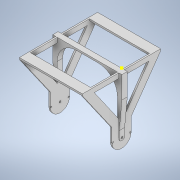
# Autodesk Inventor part: bottom_gimbal_ring_3
Saved by Autodesk Inventor 2022 (Build 260153000, 153)
## iProperties
Created: 2022-03-15
Part Number: bottom_gimbal_ring_3
Material: Generic
Document SubType Name: Modeling
Designer: kylem
Density: 1 g/cm^3
Appearance: Default
Author: kylem
Autodesk Inventor part; units mm, degrees
ref_plane "YZ Plane" through (0, 0, 0) normal (1, 0, 0) x (0, 1, 0)
ref_plane "XZ Plane" through (0, 0, 0) normal (0, 1, 0) x (-1, 0, 0)
ref_plane "XY Plane" through (0, 0, 0) normal (0, 0, 1) x (1, 0, 0)
sketch "Sketch1" plane through (0, 0, 0) normal (0, 1, 0) x (-1, 0, 0)
  circle A0 centre (0, 0) radius 16.375
  dimension "d0" = 32.75
  constraints: 1 centre point, 1 coincident
  measures "d0" diameter of A0
extrude "Extrusion1" add sketch "Sketch1" along normal blind 3
sketch "Sketch2" plane through (0, 3, 0) normal (0, 1, 0) x (1, 0, 0)
  circle A0 centre (0, 0) radius 4.75
  dimension "d3" = 9.5
  constraints: 1 centre point, 1 coincident
  measures "d3" diameter of A0
extrude "Extrusion2" add sketch "Sketch2" along normal blind 14
chamfer "Chamfer1" distance 1 angle 45 1 edges at (-4.75, 17, 0)
sketch "Sketch3" plane through (0, 3, 0) normal (0, 1, 0) x (1, 0, 0)
  circle A0 centre (0, 0) radius 15.5
  circle A1 centre (0, 0) radius 16.375
  line L0 (0, 0) -> (0, 16.375)
  circle A2 centre (0, 0) radius 16.375 projected
  line L1 (0, 0) -> (16.375, 0)
  point P0 (15.5, 0)
  point P1 (0, 15.5)
  dimension "d9" = 31
  dimension "d26" = 32.75
  constraints: 4 end point, 2 centre point, 2 coincident, 2 point on circle, 1 horizontal
  measures "d9" diameter of A0
  measures "d26" diameter of A1
extrude "Extrusion3" add sketch "Sketch3" along normal blind 13.5 contours A0 L0 A1 L1 picked at (14.8943, 5.8246)
sketch "Sketch4" plane through (0, 16.5, 0) normal (0, 1, 0) x (1, 0, 0)
  arc A0 (-10.8502, -12.2644) -> (-12.2644, -10.8502) centre (0, 0) ccw
  circle A1 centre (0, 0) radius 3.75 projected
  line L0 (0, 16.375) -> (0, 15.5) projected
  arc A2 (-10.2302, -11.6444) -> (-11.6444, -10.2302) centre (0, 0) ccw
  line L1 (0, 0) -> (-0.7071, 0.7071)
  line L2 (0, 0) -> (1, 0) construction
  line L3 (-0.7071, 0.7071) -> (0.7071, -0.7071)
  line L4 (1.0882, -0.326) -> (-18.1603, -19.5746)
  line L5 (-0.7071, 0.7071) -> (-13.3956, -11.9813)
  line L6 (-13.3956, -11.9813) -> (-11.0324, -14.3445)
  line L7 (-10.2302, -11.6444) -> (-7.7553, -14.1193)
  line L8 (-10.2302, -11.6444) -> (-6.7302, -11.6444) construction
  line L9 (-7.9511, -14.3151) -> (-11.998, -18.3619)
  line L10 (-14.4448, -7.7128) -> (-18.1483, -4.0093)
  line L11 (-11.6444, -10.2302) -> (-4.6444, -10.2302) construction
  line L12 (-18.1483, -4.0093) -> (-22.391, -8.252)
  line L13 (-18.1483, -4.0093) -> (-12.1483, -4.0093) construction
  line L14 (-13.3956, -11.9813) -> (-20.1314, -18.7172)
  line L15 (-18.1603, -19.5746) -> (-18.1603, -19.5746)
  line L16 (-18.1603, -19.5746) -> (-21.0847, -16.6502)
  line L17 (-22.391, -8.252) -> (-16.0286, -14.6144)
  line L18 (-14.4729, -15.8871) -> (-11.998, -18.3619)
  dimension "d12" = 1
  dimension "d13" = 135
  dimension "d14" = 2
  dimension "d15" = 0
  dimension "d16" = 3.5
  dimension "d17" = 45
  dimension "d18" = 6
  dimension "d19" = 90
  dimension "d20" = 9
  dimension "d21" = 135
  dimension "d22" = 6
  dimension "d23" = 135
  dimension "d29" = 16.375
  dimension "d30" = 2
  dimension "d31" = 3.5
  constraints: 36 end point, 9 perpendicular, 7 point on circle, 7 point on line, 4 horizontal, 3 equal length, 2 centre point, 2 coincident, 1 collinear
  measures "d12" distance of L1.start L1.end
  measures "d13" angle of L2 L1
  measures "d14" distance of L1.end L3.end
  measures "d15" distance between parallel lines of L3 L1
  measures "d16" distance of L7.start L7.end
  measures "d17" angle of L7 L8
  measures "d18" distance of L7.end L9.end
  measures "d19" angle of L7 L9
  measures "d20" distance of L11.start L10.end
  measures "d21" angle of L11 L10
  measures "d22" distance of L10.end L12.end
  measures "d23" angle of L12 L13
  measures "d29" radius of A0
  measures "d30" distance between parallel lines of L15 L14
  measures "d31" distance between parallel lines of L9 L4
extrude "Extrusion5" add sketch "Sketch4" against normal blind 13 contours L4 A2 L0 A0 | A0 L9 L18 L4 | L0 A2 L5 A0 | L14 L17 L12 L10 A0 L5
sketch "Sketch6" plane through (0, 16.5, 0) normal (0, 1, 0) x (1, 0, 0)
  line L0 (-11.6444, -10.2302) -> (-9.6444, -10.2302) construction
  line L1 (-22.391, -8.252) -> (-16.0286, -14.6144) projected
  line L2 (-16.0286, -14.6144) -> (-17.4428, -13.2001)
  line L3 (-16.0286, -14.6144) -> (-11.6444, -10.2302) projected
  line L4 (-16.0286, -14.6144) -> (-11.6444, -10.2302)
  line L5 (-16.0286, -14.6144) -> (-17.4428, -13.2001)
  line L6 (-16.0286, -14.6144) -> (-14.0286, -14.6144) construction
  line L7 (-17.4428, -13.2001) -> (-10.3717, -6.1291)
  line L8 (-10.3717, -6.1291) -> (-8.2504, -8.2504)
  line L9 (-10.3717, -6.1291) -> (-7.3717, -6.1291) construction
  line L10 (-8.2504, -8.2504) -> (-15.3215, -15.3215)
  line L11 (-16.0286, -14.6144) -> (-22.391, -8.252) projected
  line L12 (-15.3215, -15.3215) -> (-17.4428, -13.2001)
  line L13 (-8.252, -22.391) -> (-14.6144, -16.0286)
  line L14 (-13.2001, -17.4428) -> (-6.1291, -10.3717)
  line L15 (-6.1291, -10.3717) -> (-8.2504, -8.2504)
  line L16 (-15.3215, -15.3215) -> (-13.2001, -17.4428)
  point P0 (0, 0)
  dimension "d34" = 2
  dimension "d35" = 135
  dimension "d36" = 10
  dimension "d37" = 90
  dimension "d39" = 3
  dimension "d40" = 45
  dimension "d41" = 10
  dimension "d42" = 90
  constraints: 28 end point, 4 symmetric about line, 3 horizontal, 2 collinear, 2 equal length, 2 perpendicular, 2 point on line
  measures "d34" distance of L1.end L2.end
  measures "d35" angle of L6 L5
  measures "d36" distance of L2.end L7.end
  measures "d37" angle of L5 L7
  measures "d39" distance of L7.end L8.end
  measures "d40" angle of L8 L9
  measures "d41" distance of L8.end L10.end
  measures "d42" angle of L8 L10
extrude "Extrusion6" cut sketch "Sketch6" against normal blind 13
sketch "Sketch7" plane through (0, 16.5, 0) normal (0, 1, 0) x (1, 0, 0)
  circle A0 centre (0, 0) radius 3.75 projected
  circle A1 centre (0, 0) radius 16.375
  line L0 (-22.391, -8.252) -> (-12.1273, 2.0117)
  line L1 (-22.391, -8.252) -> (-7.876, -8.252) construction
  line L2 (-18.1483, -4.0093) -> (-14.4448, -7.7128) projected
  line L3 (-18.1483, -4.0093) -> (-14.4448, -7.7128)
  line L4 (-7.9511, -14.3151) -> (-11.998, -18.3619) projected
  line L5 (-11.998, -18.3619) -> (-9.8767, -16.2406)
  line L6 (-9.8767, -16.2406) -> (-5.4147, -15.4539)
  circle A2 centre (0, 0) radius 16.375 projected
  line L7 (-9.8767, -16.2406) -> (-7.9511, -14.3151)
  point P0 (-16.2397, -2.1007)
  dimension "d45" = 45
  dimension "d46" = 3
  dimension "d47" = 145
  constraints: 12 end point, 2 collinear, 1 centre point, 1 coincident, 1 equal length, 1 horizontal, 1 point on circle, 1 point on line
  measures "d45" angle of L1 L0
  measures "d46" distance of L4.end L5.end
  measures "d47" angle of L5 L6
extrude "Extrusion7" add sketch "Sketch7" against normal blind 13 contours L2 L0 A1 | A1 L6 L4
sketch "Sketch8" plane through (0, 16.5, 0) normal (0, 1, 0) x (1, 0, 0)
  circle A0 centre (0, 0) radius 3.75 projected
  line L0 (-13.0586, -17.3013) -> (-8.6316, -12.8742) projected
  circle A1 centre (0, 0) radius 15.5
  circle A2 centre (0, 0) radius 16.375
  arc A3 (-8.6316, -12.8742) -> (-12.8742, -8.6316) centre (0, 0) ccw projected
  circle A4 centre (0, 0) radius 27.7287
  constraints: 3 centre point, 3 coincident, 1 point on circle
extrude "Extrusion8" cut sketch "Sketch8" against normal blind 7 contours A4
chamfer "Chamfer2" distance 6 angle 45 1 edges at (-4.75, 3, 0)
sketch "Sketch9" plane through (-11.998, 3.5, 18.3619) normal (0.7071068, 0, 0.7071068) x (0.7071068, 0, -0.7071068)
  line L0 (-0.2001, 6) -> (8.4991, 6) projected
  line L1 (-0.2001, 6) -> (2.7999, 6)
  line L2 (2.7999, 6) -> (2.7999, 3)
  line L3 (3, 0) -> (3, 6) projected
  circle A0 centre (2.7999, 3) radius 1.35
  point P0 (21.4677, -3.5)
  dimension "d55" = 3
  dimension "d56" = 3
  dimension "d57" = 90
  dimension "d58" = 2.7
  constraints: 4 end point, 1 centre point, 1 coincident, 1 parallel, 1 point on line
  measures "d55" distance of L0.start L1.end
  measures "d56" distance of L1.end L2.end
  measures "d57" angle of L1 L2
  measures "d58" diameter of A0
extrude "Extrusion9" cut sketch "Sketch9" along normal mid plane 50 contours A0 L3 | A0 L3
sketch "Sketch10" plane through (-8.6316, 3.5, 12.8742) normal (-0.7071068, 0, -0.7071068) x (-0.7071068, 0, 0.7071068)
  circle A0 centre (3.4609, 3) radius 1.35 projected
  circle A1 centre (3.4609, 3) radius 1.6
  point P0 (-15.2069, -3.5)
  dimension "d61" = 3.2
  constraints: 1 centre point, 1 coincident
  measures "d61" diameter of A1
extrude "Extrusion10" cut sketch "Sketch10" against normal blind 50 contours A0 | A1
sketch "Sketch11" plane through (-11.998, 3.5, 18.3619) normal (0.7071068, 0, 0.7071068) x (0.7071068, 0, -0.7071068)
  arc A0 (3, 1.4126) -> (3, 4.5874) centre (2.7999, 3) ccw projected
  circle A1 centre (2.7999, 3) radius 3
  line L0 (3, 0) -> (0, 0) projected
  point P0 (21.4677, -3.5)
  constraints: 1 centre point, 1 coincident, 1 tangent
extrude "Extrusion11" cut sketch "Sketch11" along normal blind 50
sketch "Sketch12" plane through (0, 16.5, 0) normal (0, 1, 0) x (1, 0, 0)
  circle A0 centre (0, 0) radius 3.75 projected
  arc A1 (-9.2616, -13.5042) -> (-13.5042, -9.2616) centre (0, 0) ccw
  arc A2 (-9.5312, -13.7738) -> (-13.7738, -9.5312) centre (0, 0) ccw
  arc A3 (-8.6316, -12.8742) -> (-12.8742, -8.6316) centre (0, 0) ccw projected
  line L0 (-17.4428, -13.2001) -> (-22.391, -8.252) projected
  line L1 (-12.8742, -8.6316) -> (-17.4428, -13.2001)
  line L2 (-13.0586, -17.3013) -> (-8.6316, -12.8742) projected
  line L3 (-8.6316, -12.8742) -> (-13.0586, -17.3013)
  point P0 (-9.2616, -13.5042)
  dimension "d66" = 33.5
  constraints: 4 end point, 4 point on circle, 4 point on line, 2 centre point, 2 coincident, 1 collinear, 1 perpendicular
  measures "d66" diameter of A2
extrude "Extrusion12" add sketch "Sketch12" against normal blind 13 contours A1 L1 A2 L2
sketch "Sketch13" plane through (0, 3.5, 0) normal (0, -1, 0) x (1, 0, 0)
  circle A0 centre (0, 0) radius 16.75
  arc A1 (-13.7738, 9.5312) -> (-9.5312, 13.7738) centre (0, 0) ccw projected
  line L0 (0, -15.5) -> (0, -16.375) projected
  circle A2 centre (0, 0) radius 16.375
  line L1 (0, 0) -> (0, -16.75)
  line L2 (0, 0) -> (16.75, 0)
  point P0 (16.75, 0)
  point P1 (16.375, 0)
  constraints: 4 end point, 2 coincident, 2 point on circle, 1 centre point, 1 perpendicular, 1 vertical, 3 other
extrude "Extrusion13" add sketch "Sketch13" along normal blind 3.5 contours A0 L1 A2 L2 picked at (2.457, -16.3482)
sketch "Sketch14" plane through (0, 0, 0) normal (0, -1, 0) x (1, 0, 0)
  line L0 (0, -16.375) -> (0, -16.75) projected
  circle A0 centre (0, 0) radius 16.75
  constraints: 1 coincident, 1 vertical alignment, 2 other
extrude "Extrusion14" add sketch "Sketch14" against normal blind 3
sketch "Sketch18" plane through (0, 0, 0) normal (0, 0, 1) x (1, 0, 0)
  line L0 (0, 0) -> (-78.5, 0)
  line L1 (-16.75, 0) -> (16.75, 0) projected
  line L2 (-78.5, 0) -> (78.5, 0)
  line L3 (78.5, 0) -> (78.5, -12)
  line L4 (-78.5, -12) -> (-78.5, 0)
  line L5 (-78.5, -157) -> (78.5, -157)
  line L6 (78.5, -157) -> (90.5, -157)
  line L7 (90.5, -157) -> (90.5, 0)
  line L8 (90.5, 0) -> (78.5, 0)
  line L9 (-78.5, -157) -> (-90.5, -157)
  line L10 (-90.5, -157) -> (-90.5, 0)
  line L11 (-90.5, 0) -> (-78.5, 0)
  line L12 (-78.5, -12) -> (-65.1606, -12)
  line L13 (-28.5, -12) -> (-28.5, -62)
  line L14 (-28.5, -62) -> (-78.5, -62)
  line L15 (-78.5, -25.3394) -> (-78.5, -12)
  line L16 (78.5, -12) -> (65.1606, -12)
  line L17 (28.5, -12) -> (28.5, -62)
  line L18 (28.5, -62) -> (78.5, -62)
  line L19 (78.5, -25.3394) -> (78.5, -12)
  circle A0 centre (28.5, -62) radius 50
  circle A1 centre (-28.5, -62) radius 50
  line L20 (78.5, -157) -> (78.5, -62)
  line L21 (78.5, -25.3394) -> (78.5, -12)
  line L22 (78.5, -12) -> (65.1606, -12)
  arc A2 (90.5, -62) -> (28.5, 0) centre (28.5, -62) ccw
  arc A3 (-8.1606, -12) -> (78.5, -98.6606) centre (28.5, -62) ccw
  line L23 (-78.5, -12) -> (-78.5, -25.3394)
  line L24 (-78.5, -62) -> (-78.5, -157)
  line L25 (-65.1606, -12) -> (-78.5, -12)
  line L26 (28.5, -12) -> (-28.5, -12)
  line L27 (-65.1606, -12) -> (-78.5, -12)
  line L28 (-78.5, 0) -> (-78.5, -25.3394)
  line L29 (-78.5, -62) -> (-78.5, -157)
  arc A4 (-28.5, 0) -> (-90.5, -62) centre (-28.5, -62) ccw
  arc A5 (-78.5, -98.6606) -> (8.1606, -12) centre (-28.5, -62) ccw
  line L30 (78.5, 0) -> (78.5, -25.3394)
  line L31 (78.5, -62) -> (78.5, -157)
  line L32 (78.5, -12) -> (65.1606, -12)
  line L33 (28.5, -12) -> (-28.5, -12)
  dimension "d82" = 78.5
  dimension "d83" = 157
  dimension "d84" = 12
  dimension "d85" = 157
  dimension "d86" = 145
  dimension "d87" = 12
  dimension "d88" = 157
  dimension "d89" = 12
  dimension "d90" = 157
  dimension "d91" = 50
  dimension "d92" = 50
  dimension "d93" = 50
  dimension "d94" = 50
  constraints: 66 end point, 21 parallel, 12 point on circle, 11 perpendicular, 8 horizontal, 8 point on line, 4 centre point, 4 coincident, 1 collinear, 6 other
  measures "d82" distance of L0.start L0.end
  measures "d83" distance of L3.end L4.start
  measures "d84" distance of L2.end L3.end
  measures "d85" distance of L5.end L5.start
  measures "d86" distance of L5.start L12.start
  measures "d87" distance of L8.end L7.end
  measures "d88" distance of L7.end L6.end
  measures "d89" distance of L10.end L11.end
  measures "d90" distance of L9.end L10.end
  measures "d91" distance of L13.end L14.end
  measures "d92" distance of L13.start L13.end
  measures "d93" distance of L18.end L17.end
  measures "d94" distance of L17.start L17.end
extrude "Extrusion16" add sketch "Sketch18" along normal mid plane 14 contours L1 L2 A2 L7 L6 L20 A0 L26 A1 L24 L9 L10 A4 L0
sketch "Sketch19" plane through (90.5, -157, 7) normal (1, 0, 0) x (0, 0, -1)
  line L0 (14, 0) -> (0, 0) projected
  line L1 (0, 0) -> (0, 95) projected
  circle A0 centre (7, 0) radius 7
  point P0 (7, 157)
  constraints: 1 midpoint, 3 other
extrude "Extrusion17" add sketch "Sketch19" against normal blind 12 contours A0 L0 picked at (9.1339, -1.6428)
ref_plane "Work Plane1" through (0, -62, -7) normal (-1, 0, 0) x (0, 0, 1)
mirror "Mirror1" about plane through (0, -62, -7) normal (-1, 0, 0) of "Extrusion17"
sketch "Sketch20" plane through (90.5, -62, 7) normal (1, 0, 0) x (0, 0, -1)
  arc A0 (0, -95) -> (14, -95) centre (7, -95) ccw projected
  circle A1 centre (7, -95) radius 4.125
  point P0 (7, 62)
  dimension "d101" = 8.25
  constraints: 1 centre point, 1 coincident
  measures "d101" diameter of A1
extrude "Extrusion18" cut sketch "Sketch20" against normal blind 200
sketch "Sketch21" plane through (0, 0, 7) normal (0, 0, 1) x (1, 0, 0)
  line L0 (78.5, -157) -> (78.5, -62) projected
  line L1 (78.5, -157) -> (82.5, -157)
  line L2 (82.5, -157) -> (82.5, -148)
  line L3 (82.5, -148) -> (78.5, -148)
  line L4 (78.5, -148) -> (78.5, -157)
  line L5 (78.5, -157) -> (78.5, -164) projected
  line L6 (78.5, -164) -> (82.5, -164)
  line L7 (82.5, -164) -> (82.5, -157)
  line L8 (82.5, -157) -> (78.5, -157)
  line L9 (78.5, -157) -> (78.5, -164)
  line L10 (90.5, -164) -> (90.5, -157) projected
  line L11 (90.5, -164) -> (82.5, -164)
  line L12 (82.5, -164) -> (82.5, -148)
  line L13 (82.5, -148) -> (90.5, -148)
  line L14 (90.5, -148) -> (90.5, -164)
  point P0 (0, 0)
  dimension "d104" = 4
  dimension "d105" = 9
  constraints: 24 end point, 6 parallel, 3 horizontal, 3 perpendicular
  measures "d104" distance of L3.end L2.end
  measures "d105" distance of L2.end L1.end
extrude "Extrusion19" cut sketch "Sketch21" against normal blind 200 contours L2 L13 L14 L10 L11 L7
mirror "Mirror2" about plane through (0, -62, -7) normal (-1, 0, 0) of "Extrusion19"
chamfer "Chamfer3" distance 8 angle 84.5 1 edges at (90.5, -148, 0) measured on face at (90, -148, 0)
chamfer "Chamfer4" distance 8 angle 84.5 1 edges at (-90.5, -148, 0) measured on face at (-90, -148, 0)
sketch "Sketch22" plane through (82.5, -157, 0) normal (1, 0, 0) x (0, 0, -1)
  line L0 (0, 0) -> (-0.3, 0)
  line L1 (-0.3, 0) -> (0.3, 0)
  line L2 (0.3, 0) -> (0.3, -10.622)
  line L3 (0.3, -10.622) -> (-0.3, -10.622)
  line L4 (-0.3, -10.622) -> (-0.3, 0)
  arc A0 (-7, 0) -> (7, 0) centre (0, 0) ccw projected
  line L5 (0, -7) -> (0, -6)
  line L6 (0, -6) -> (-0.3, -6)
  line L7 (-0.3, -6) -> (0.3, -6)
  point P0 (0, 157)
  point P1 (0, -6)
  point P2 (-0.3, -6.9936)
  point P3 (0.3, -6.9936)
  dimension "d117" = 0.3
  dimension "d118" = 0.6
  dimension "d119" = 1
  constraints: 16 end point, 3 point on line, 2 horizontal, 2 parallel, 2 perpendicular, 1 point on circle, 1 vertical
  measures "d117" distance of L0.start L0.end
  measures "d118" distance of L2.end L3.end
  measures "d119" distance of L5.start L5.end
extrude "Extrusion20" cut sketch "Sketch22" against normal blind 1200 contours L6 L5 A0 L4 | L2 A0 L5 L7
sketch "Sketch23" plane through (0, 17, 0) normal (0, 1, 0) x (1, 0, 0)
  circle A0 centre (0, 0) radius 3.75 projected
  circle A1 centre (0, 0) radius 37.5
  dimension "d124" = 75
  constraints: 1 centre point, 1 coincident
  measures "d124" diameter of A1
extrude "Extrusion22" cut sketch "Sketch23" against normal blind 20 contours A0 | A1
sketch "Sketch24" plane through (0, -3, 0) normal (0, 1, 0) x (1, 0, 0)
  circle A0 centre (0, 0) radius 100
  dimension "d127" = 200
  constraints: 1 centre point, 1 coincident
  measures "d127" diameter of A0
extrude "Extrusion23" cut sketch "Sketch24" along normal mid plane 16
sketch "Sketch27" plane through (0, -11, 0) normal (0, 1, 0) x (1, 0, 0)
  circle A0 centre (0, 0) radius 100
  dimension "d141" = 200
  constraints: 1 centre point, 1 coincident
  measures "d141" diameter of A0
extrude "Extrusion26" add sketch "Sketch27" along normal blind 3.5
sketch "Sketch28" plane through (0, -11, 0) normal (0, -1, 0) x (1, 0, 0)
  circle A0 centre (0, 0) radius 100
  constraints: 1 centre point, 1 coincident
extrude "Extrusion27" add sketch "Sketch28" along normal blind 1
ref_plane "Work Plane2" through (-90.5, -64.9168, -3) normal (-1, 0, 0) x (0, 0, 1)
sketch "Sketch30" plane through (-90.5, -62, -7) normal (-1, 0, 0) x (0, 0, 1)
  line L0 (0, 0) -> (14, 0) projected
  line L1 (0, 50) -> (14, 50) projected
  line L2 (14, 0) -> (0, 0)
  line L3 (0, 0) -> (0, 50)
  line L4 (0, 50) -> (14, 50)
  line L5 (14, 50) -> (14, 0)
  point P0 (7, 62)
  constraints: 8 end point, 2 parallel, 1 horizontal, 1 perpendicular
extrude "Extrusion29" cut sketch "Sketch30" against normal blind 200
sketch "Sketch31" plane through (-90.5, -62, 7) normal (0, 1, 0) x (1, 0, 0)
  line L0 (0, 0) -> (0, 14) projected
  line L1 (12, 0) -> (0, 0)
  line L2 (0, 0) -> (0, 14)
  line L3 (0, 14) -> (12, 14)
  line L4 (12, 14) -> (12, 0)
  line L5 (181, 14) -> (181, 0) projected
  line L6 (169, 0) -> (181, 0)
  line L7 (181, 0) -> (181, 14)
  line L8 (181, 14) -> (169, 14)
  line L9 (169, 14) -> (169, 0)
  point P0 (90.5, 7)
  constraints: 16 end point, 4 parallel, 2 horizontal, 2 perpendicular
extrude "Extrusion30" add sketch "Sketch31" along normal blind 50
fillet "Fillet1" radius 50 2 edges at (-78.5, -12, 0) (78.5, -12, 0)
sketch "Sketch33" plane through (-78.5, -157, 7) normal (1, 0, 0) x (0, 0, -1)
  line L0 (0, 95) -> (14, 95) projected
  line L1 (14, 95) -> (14, 55)
  line L2 (14, 0) -> (14, 95) projected
  line L3 (14, 55) -> (107.8943, 231.5895)
  line L4 (14, 55) -> (14, 145)
  line L5 (-93, 145) -> (107, 145) projected
  line L6 (0, 145) -> (14, 145) projected
  line L7 (14, 145) -> (61.8538, 145)
  point P0 (7, 157)
  point P1 (61.8538, 145)
  dimension "d153" = 40
  dimension "d154" = 200
  dimension "d155" = 28
  constraints: 8 end point, 3 point on line, 1 collinear, 1 vertical
  measures "d153" distance of L0.end L1.end
  measures "d154" distance of L1.end L3.end
  measures "d155" angle of L3 L1
extrude "Extrusion31" add sketch "Sketch33" against normal blind 4
ref_plane "Work Plane3" through (0, 0, 0) normal (0, 0, -1) x (-1, 0, 0)
ref_plane "Work Plane4" through (0, -157, -7) normal (-1, 0, 0) x (0, 0, 1)
mirror "Mirror3" about plane through (0, 0, 0) normal (0, 0, -1) of "Extrusion31"
mirror "Mirror4" about plane through (0, -157, -7) normal (-1, 0, 0) of "Extrusion31", "Mirror3"
sketch "Sketch34" plane through (0, -12, 0) normal (0, -1, 0) x (1, 0, 0)
  line L0 (90.5, -7) -> (90.5, 7) projected
  line L1 (90.5, -7) -> (108.0543, -7)
  line L2 (108.0543, -7) -> (108.0543, -67.2523)
  line L3 (108.0543, -67.2523) -> (90.5, -67.2523)
  line L4 (90.5, -67.2523) -> (90.5, -7)
  line L5 (90.5, -7) -> (110.0545, -7)
  line L6 (110.0545, -7) -> (110.0545, 70.2775)
  line L7 (110.0545, 70.2775) -> (90.5, 70.2775)
  line L8 (90.5, 70.2775) -> (90.5, -7)
  line L9 (-90.5, 7) -> (-90.5, -7) projected
  line L10 (-90.5, -7) -> (-103.7572, -7)
  line L11 (-103.7572, -7) -> (-103.7572, -108.2386)
  line L12 (-103.7572, -108.2386) -> (-90.5, -108.2386)
  line L13 (-90.5, -108.2386) -> (-90.5, -7)
  line L14 (-90.5, -7) -> (-103.7572, -7)
  line L15 (-103.7572, -7) -> (-103.7572, 99.0549)
  line L16 (-103.7572, 99.0549) -> (-90.5, 99.0549)
  line L17 (-90.5, 99.0549) -> (-90.5, -7)
  point P0 (0, 0)
  constraints: 32 end point, 8 parallel, 4 horizontal, 4 perpendicular, 1 point on line
extrude "Extrusion32" cut sketch "Sketch34" against normal blind 34
sketch "Sketch35" plane through (0, -12, 0) normal (0, -1, 0) x (1, 0, 0)
  line L0 (-82.5, 7) -> (-90.5, 7) projected
  line L1 (-82.5, 7) -> (-95.4434, 7)
  line L2 (-95.4434, 7) -> (-95.4434, 67.1628)
  line L3 (-95.4434, 67.1628) -> (-82.5, 67.1628)
  line L4 (-82.5, 67.1628) -> (-82.5, 7)
  line L5 (-82.5, -54.8538) -> (-82.5, -7) projected
  line L6 (-82.5, -7) -> (-99.6148, -7)
  line L7 (-99.6148, -7) -> (-99.6148, -59.6293)
  line L8 (-99.6148, -59.6293) -> (-82.5, -59.6293)
  line L9 (-82.5, -59.6293) -> (-82.5, -7)
  line L10 (82.5, 7) -> (90.5, 7) projected
  line L11 (82.5, 7) -> (108.5087, 7)
  line L12 (108.5087, 7) -> (108.5087, 67.857)
  line L13 (108.5087, 67.857) -> (82.5, 67.857)
  line L14 (82.5, 67.857) -> (82.5, 7)
  line L15 (82.5, -7) -> (82.5, -54.8538) projected
  line L16 (82.5, -7) -> (100.3629, -7)
  line L17 (100.3629, -7) -> (100.3629, -69.6425)
  line L18 (100.3629, -69.6425) -> (82.5, -69.6425)
  line L19 (82.5, -69.6425) -> (82.5, -7)
  point P0 (0, 0)
  constraints: 32 end point, 8 parallel, 4 horizontal, 4 perpendicular
extrude "Extrusion33" cut sketch "Sketch35" against normal blind 34
sketch "Sketch36" plane through (-78.5, -62, 7) normal (1, 0, 0) x (0, 0, -1)
  line L0 (0, -86) -> (14, -86) projected
  line L1 (14, -86) -> (128.7153, 77.8304)
  line L2 (14, -86) -> (214, -86) construction
  line L3 (14, 50) -> (14, -86)
  line L4 (14, -95) -> (14, -40) projected
  line L5 (-49.5133, 54.5) -> (-93, 54.5) projected
  line L6 (-49.5133, 54.5) -> (170.0067, 54.5)
  line L7 (14, 54.5) -> (14, -40) projected
  line L8 (14, -86) -> (14, 54.5)
  line L9 (14, 54.5) -> (112.3792, 54.5)
  line L10 (14, -95) -> (14, -86) projected
  line L11 (112.3792, 54.5) -> (14, -86)
  point P0 (7, 62)
  point P1 (63.5133, 50)
  dimension "d162" = 200
  dimension "d163" = 55
  constraints: 14 end point, 4 point on line, 2 horizontal, 1 collinear, 1 equal length
  measures "d162" distance of L0.end L1.end
  measures "d163" angle of L2 L1
extrude "Extrusion34" add sketch "Sketch36" against normal blind 4
mirror "Mirror5" about plane through (0, 0, 0) normal (0, 0, 1) of "Extrusion34"
mirror "Mirror6" about plane through (0, 0, 0) normal (1, 0, 0) of "Extrusion34", "Mirror5"
sketch "Sketch37" plane through (0, -7.5, 0) normal (0, 1, 0) x (1, 0, 0)
  line L0 (-82.5, 105.3792) -> (-82.5, 7) projected
  line L1 (78.5, -105.3792) -> (82.5, -105.3792) projected
  line L2 (-82.5, 105.3792) -> (82.5, 105.3792)
  line L3 (82.5, 105.3792) -> (82.5, -105.3792)
  line L4 (82.5, -105.3792) -> (-82.5, -105.3792)
  line L5 (-82.5, -105.3792) -> (-82.5, 105.3792)
  point P0 (0, 0)
  point P1 (-82.5, 7)
  constraints: 8 end point, 2 parallel, 1 horizontal, 1 perpendicular
extrude "Extrusion35" add sketch "Sketch37" against normal blind 4.5
sketch "Sketch38" plane through (-78.5, -12, 7) normal (0, -1, 0) x (1, 0, 0)
  line L0 (0, 95.2282) -> (-4, 95.2282) projected
  line L1 (161, 0) -> (161, 98.3792) projected
  line L2 (-4, 95.2282) -> (161, 95.2282)
  line L3 (161, 95.2282) -> (161, 98.3792)
  line L4 (161, 98.3792) -> (-4, 98.3792)
  line L5 (-4, 98.3792) -> (-4, 95.2282)
  line L6 (161, -112.3792) -> (161, -109.2282) projected
  line L7 (-4, -109.2282) -> (-4, -112.3792) projected
  line L8 (161, -109.2282) -> (-4, -109.2282)
  line L9 (-4, -109.2282) -> (-4, -112.3792)
  line L10 (-4, -112.3792) -> (161, -112.3792)
  line L11 (161, -112.3792) -> (161, -109.2282)
  point P0 (78.5, -7)
  constraints: 16 end point, 4 parallel, 2 horizontal, 2 perpendicular
extrude "Extrusion36" cut sketch "Sketch38" against normal blind 4.5
sketch "Sketch39" plane through (82.5, -148, -7) normal (1, 0, 0) x (0, 0, -1)
  line L0 (0, 83.0832) -> (0, 140.5) projected
  line L1 (0, 140.5) -> (0, 136)
  line L2 (0, 136) -> (0, 36)
  line L3 (0, 0) -> (0, 140.5) projected
  line L4 (0, 36) -> (74.5649, 142.4898)
  line L5 (0, 36) -> (130, 36) construction
  line L6 (0, 136) -> (124.2806, 136)
  line L7 (0, 36) -> (0, 170.1801)
  line L8 (0, 136) -> (109.9914, 136)
  line L9 (74.5649, 142.4898) -> (-35.3209, -14.4435)
  point P0 (-7, 148)
  point P1 (70.0208, 136)
  dimension "d170" = 4.5
  dimension "d171" = 100
  dimension "d172" = 130
  dimension "d173" = 55
  constraints: 16 end point, 4 point on line, 2 horizontal, 1 equal length
  measures "d170" distance of L0.end L1.end
  measures "d171" distance of L1.end L2.end
  measures "d172" distance of L2.end L4.end
  measures "d173" angle of L5 L4
extrude "Extrusion37" cut sketch "Sketch39" along normal mid plane 400
mirror "Mirror7" about plane through (0, 0, 0) normal (0, 0, 1) of "Extrusion37"
sketch "Sketch40" plane through (-28.5, -12, -7) normal (0, -1, 0) x (1, 0, 0)
  line L0 (-54, -70.0208) -> (-50, -70.0208) projected
  line L1 (-50, -70.0208) -> (129.2455, -70.0208)
  line L2 (107, 0) -> (107, -70.0208) projected
  line L3 (-50, -70.0208) -> (107, -70.0208)
  line L4 (107, -70.0208) -> (107, 0)
  line L5 (107, 0) -> (-50, 0)
  line L6 (-50, 0) -> (-50, -70.0208)
  point P0 (28.5, 7)
  constraints: 10 end point, 2 horizontal, 2 parallel, 1 perpendicular
extrude "Extrusion38" cut sketch "Sketch40" against normal blind 10
sketch "Sketch43" plane through (-82.5, -12, -77.0208) normal (0, -1, 0) x (1, 0, 0)
  line L0 (4, 0) -> (161, 0) projected
  line L1 (0, 84.0208) -> (0, 70.0208) projected
  line L2 (4, 0) -> (0, 0)
  line L3 (0, 0) -> (0, 70.0208)
  line L4 (0, 70.0208) -> (4, 70.0208)
  line L5 (4, 70.0208) -> (4, 0)
  line L6 (161, 70.0208) -> (161, -25.2075) projected
  line L7 (165, 70.0208) -> (165, -25.2075) projected
  line L8 (161, 0) -> (165, 0)
  line L9 (165, 0) -> (165, 70.0208)
  line L10 (165, 70.0208) -> (161, 70.0208)
  line L11 (161, 70.0208) -> (161, 0)
  point P0 (82.5, 77.0208)
  constraints: 16 end point, 4 parallel, 2 horizontal, 2 perpendicular, 2 point on line
extrude "Extrusion41" add sketch "Sketch43" along normal blind 8
mirror "Mirror8" about plane through (0, 0, 0) normal (0, 0, 1) of "Extrusion38", "Extrusion41"
sketch "Sketch44" plane through (-78.5, -62, 7) normal (1, 0, 0) x (0, 0, -1)
  circle A0 centre (7, -95) radius 4.125 projected
  circle A1 centre (7, -95) radius 25
  point P0 (7, 62)
  dimension "d185" = 50
  constraints: 1 centre point, 1 coincident
  measures "d185" diameter of A1
extrude "Extrusion42" add sketch "Sketch44" against normal blind 5
sketch "Sketch45" plane through (-83.5, -62, 7) normal (-1, 0, 0) x (0, 0, 1)
  circle A0 centre (-7, -95) radius 4.125 projected
  circle A1 centre (-7, -95) radius 2.55
  point P0 (-7, 62)
  dimension "d188" = 5.1
  constraints: 1 centre point, 1 coincident
  measures "d188" diameter of A1
extrude "Extrusion43" add sketch "Sketch45" against normal blind 5
sketch "Sketch46" plane through (-83.5, -62, 7) normal (-1, 0, 0) x (0, 0, 1)
  circle A0 centre (-7, -95) radius 2.55 projected
  circle A1 centre (-7, -95) radius 25
  line L0 (-7, -95) -> (18, -95)
  arc A2 (-21.8041, -74.8546) -> (7.8041, -74.8546) centre (-7, -95) ccw projected
  line L1 (18, -95) -> (15.5, -95)
  circle A3 centre (15.5, -95) radius 1.65
  arc A4 (-14, -95) -> (-7.3, -101.9936) centre (-7, -95) ccw projected
  line L2 (-7, -95) -> (-7, -107.1097)
  circle A5 centre (-29.5, -95) radius 1.65
  point P0 (-7, 62)
  dimension "d191" = 2.5
  dimension "d192" = 3.3
  constraints: 6 end point, 3 centre point, 2 coincident, 1 horizontal, 1 point on circle, 1 point on line, 1 symmetric about line, 1 vertical, 1 other
  measures "d191" distance of L0.end L1.end
  measures "d192" diameter of A3
extrude "Extrusion44" cut sketch "Sketch46" against normal blind 5 contours L0 A3 | L0 A3 | A5
mirror "Mirror9" about plane through (0, 0, 0) normal (1, 0, 0) of "Extrusion42", "Extrusion43", "Extrusion44"
sketch "Sketch47" plane through (-78.5, -62, 7) normal (1, 0, 0) x (0, 0, -1)
  arc A0 (0, -71) -> (14, -71) centre (7, -95) ccw projected
  line L0 (32, -95) -> (32, -57.5628)
  line L1 (21.8041, -74.8546) -> (109.2282, 50) projected
  line L2 (21.8041, -74.8546) -> (36.4826, -53.8915)
  circle A1 centre (7, -95) radius 25
  circle A2 centre (7, -95) radius 2.55 projected
  line L3 (7, -95) -> (7, -85.7094)
  arc A3 (0, -71) -> (14, -71) centre (7, -95) ccw
  line L4 (-18, -95) -> (-18, -57.5628)
  line L5 (-7.8041, -74.8546) -> (-95.2282, 50)
  point P0 (7, 62)
  point P1 (-7.8041, -74.8546)
  point P2 (-18, -60.2933)
  point P3 (32, -60.2933)
  constraints: 10 end point, 6 symmetric about line, 4 point on circle, 2 centre point, 2 vertical, 1 coincident, 1 point on line, 1 tangent, 1 other
extrude "Extrusion45" add sketch "Sketch47" against normal blind 5 contours A0 L4 L5 | L1 L0 A0
mirror "Mirror10" about plane through (0, 0, 0) normal (1, 0, 0) of "Extrusion45"
sketch "Sketch48" plane through (-83.5, -62, 7) normal (-1, 0, 0) x (0, 0, 1)
  circle A0 centre (-7, -95) radius 2.55 projected
  circle A1 centre (-7, -95) radius 7
  arc A2 (7.8041, -74.8546) -> (0, -71) centre (-7, -95) ccw projected
  circle A3 centre (-7, -95) radius 25
  line L0 (18, -60.2933) -> (95.2282, 50) projected
  line L1 (-7, -95) -> (18, -60.2933)
  line L2 (18, -60.2933) -> (18, -95) projected
  line L3 (18, -60.2933) -> (18, -95)
  line L4 (-32, -95) -> (-32, -60.2933) projected
  line L5 (-32, -95) -> (-32, -60.2933)
  line L6 (-32, -60.2933) -> (-21.8041, -74.8546)
  line L7 (-32, -60.2933) -> (-109.2282, 50) projected
  line L8 (-14, -75.6146) -> (-14, -2.9168) projected
  line L9 (-14, -71) -> (-14, -95)
  line L10 (0, -95) -> (0, -71)
  line L11 (0, -2.9168) -> (0, -75.6146) projected
  point P0 (-7, 62)
  point P1 (7.6119, -74.7147)
  dimension "d221" = 14
  constraints: 12 end point, 5 point on circle, 4 collinear, 2 centre point, 2 coincident, 2 tangent, 1 point on line
  measures "d221" diameter of A1
extrude "Extrusion46" cut sketch "Sketch48" against normal blind 1 contours A1 L10 L1 A2 A3 L8 L9 | L10 A2 L1 | L1 L2 A3 A2 | A3 L4 L6
mirror "Mirror11" about plane through (0, 0, 0) normal (1, 0, 0) of "Extrusion46"
sketch "Sketch49" plane through (82.5, -7.5, 102.2282) normal (1, 0, 0) x (0, 0, -1)
  point P0 (102.2282, 7.5)
body "Solid1"
